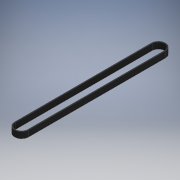
# Autodesk Inventor part: 皮带
Saved by Autodesk Inventor 2017 (Build 210142000, 142)
## iProperties
Part Number: 皮带
Material: 常规
Document SubType Name: Modeling
Designer: PANDA
Density: 1 g/cm^3
Appearance: 默认
Author: PANDA
Autodesk Inventor part; units mm, degrees
ref_plane "YZ Plane" through (0, 0, 0) normal (1, 0, 0) x (0, 1, 0)
ref_plane "XZ Plane" through (0, 0, 0) normal (0, 1, 0) x (-1, 0, 0)
ref_plane "XY Plane" through (0, 0, 0) normal (0, 0, 1) x (1, 0, 0)
sketch "草图5" plane through (0, 0, 0) normal (0, 0, 1) x (1, 0, 0)
  line L0 (0, 0) -> (0, 450) construction
  line L1 (20, 0) -> (20, 450)
  line L2 (-20, 450) -> (-20, 0)
  arc A0 (-20, 0) -> (20, 0) centre (0, 0) ccw
  arc A1 (20, 450) -> (-20, 450) centre (0, 450) ccw
  line L3 (0, 0) -> (450, 0) construction
  line L4 (0, 0) -> (0, 450) construction
  line L5 (23, 0) -> (23, 450)
  line L6 (-23, 450) -> (-23, 0)
  arc A2 (-23, 0) -> (23, 0) centre (0, 0) ccw
  arc A3 (23, 450) -> (-23, 450) centre (0, 450) ccw
  line L7 (0, 0) -> (450, 0) construction
  point P0 (0, 225)
  point P1 (0, 225)
  dimension "d23" = 450
  dimension "d24" = 90
  dimension "d25" = 40
  dimension "d26" = 450
  dimension "d27" = 90
  dimension "d28" = 46
  constraints: 20 end point, 8 point on circle, 8 tangent, 4 centre point, 3 parallel, 2 horizontal, 2 midpoint, 2 perpendicular, 1 vertical
  measures "d23" distance of L0.start L0.end
  measures "d24" angle of L3 L0
  measures "d25" diameter of A1
  measures "d26" distance of L0.start L0.end
  measures "d27" angle of L7 L4
  measures "d28" diameter of A3
extrude "拉伸4" add sketch "草图5" along normal blind 20
